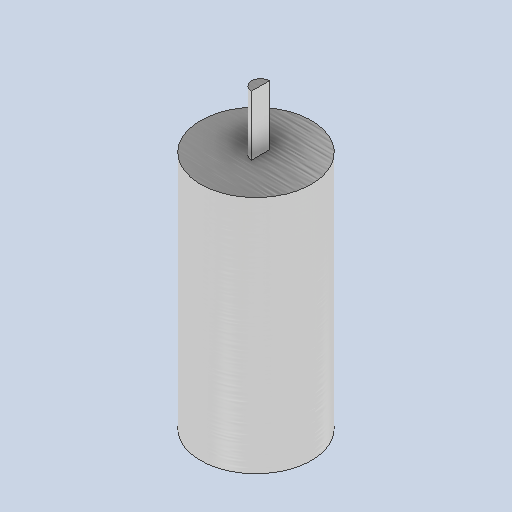
# Autodesk Inventor part: motor
Saved by Autodesk Inventor 2025.3 (Build 293356030, 356C)
## iProperties
Created: 2026-06-25
Part Number: motor
Material: Generic
Document SubType Name: Modeling
Designer: user
Density: 1 g/cm^3
Appearance: Chrome - Polished Brushed
Author: user
Autodesk Inventor part; units mm, degrees
ref_plane "YZ Plane" through (0, 0, 0) normal (1, 0, 0) x (0, 1, 0)
ref_plane "XZ Plane" through (0, 0, 0) normal (0, 1, 0) x (-1, 0, 0)
ref_plane "XY Plane" through (0, 0, 0) normal (0, 0, 1) x (1, 0, 0)
sketch "Sketch1" plane through (0, 0, 0) normal (0, 1, 0) x (-1, 0, 0)
  circle A0 centre (0, 0) radius 18.5
  arc A1 (-1.5, -3) -> (-1.5, 3) centre (-1.5, 0) ccw
  line L0 (-1.5, 0) -> (-1.5, -3) construction
  line L1 (-1.5, 0) -> (1.5, 0) construction
  line L2 (-1.5, 0) -> (-1.5, 3) construction
  line L3 (-1.5, 3) -> (-1.5, -3)
  dimension "d4" = 3
  dimension "d6" = 37
  constraints: 8 end point, 3 point on circle, 2 centre point, 1 coincident, 1 horizontal, 1 perpendicular
  measures "d4" radius of A1
  measures "d6" diameter of A0
extrude "Extrusion1" add sketch "Sketch1" along normal blind 20 contours L3 A1
extrude "Extrusion2" add sketch "Sketch1" against normal blind 80
body "Solid1"
